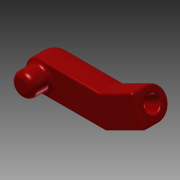
# Autodesk Inventor part: Lego Arm
Saved by Autodesk Inventor 2013 (Build 170138000, 138)
## iProperties
Created: 2013-09-06
Part Number: Lego Arm
Material: Generic
Document SubType Name: Modeling
Designer: 200395375
Density: 1 g/cm^3
Mass: 0.228717 g
Surface Area: 2.72541 cm^2
Volume: 0.228717 cm^3
Author: 200395375
Autodesk Inventor part; units mm, degrees
ref_plane "YZ Plane" through (0, 0, 0) normal (1, 0, 0) x (0, 1, 0)
ref_plane "XZ Plane" through (0, 0, 0) normal (0, 1, 0) x (-1, 0, 0)
ref_plane "XY Plane" through (0, 0, 0) normal (0, 0, 1) x (1, 0, 0)
sketch "Sketch16" plane through (0, 0, 0) normal (0, 1, 0) x (-1, 0, 0)
  circle A0 centre (0, 0) radius 1.5
  dimension "d51" = 3
  constraints: 1 centre point, 1 coincident
  measures "d51" diameter of A0
extrude "Extrusion15" add sketch "Sketch16" along normal blind 2.5
sketch "Sketch17" plane through (0, 2.5, 0) normal (0, 1, 0) x (1, 0, 0)
  line L0 (2, 2) -> (-2, 2)
  line L1 (-2, 2) -> (-2, -2)
  line L2 (-2, -2) -> (2, -2)
  line L3 (2, -2) -> (2, 2)
  dimension "d54" = 4
  dimension "d55" = 4
  constraints: 8 end point, 2 parallel, 1 horizontal, 1 perpendicular
  measures "d54" distance of L2.end L1.end
  measures "d55" distance of L1.end L0.end
extrude "Extrusion16" add sketch "Sketch17" along normal blind 4
sketch "Sketch18" plane through (2, 2.5, 2) normal (1, 0, 0) x (0, 0, -1)
  line L0 (0, 0) -> (4, 0) projected
  line L1 (4, 0) -> (4, 4) projected
  line L2 (0, 4) -> (4, 4) projected
  line L3 (0, 0) -> (0, 4) projected
  point P0 (2, -2.5)
extrude "Extrusion17" add sketch "Sketch18" along normal blind 6
sketch "Sketch21" plane through (0, 6.5, 0) normal (0, 1, 0) x (1, 0, 0)
  line L0 (8, 2) -> (8, -2) projected
  line L1 (8, 2) -> (10, 2)
  line L2 (10, 2) -> (8, -2)
  point P0 (0, 0)
  dimension "d66" = 2
  constraints: 4 end point, 1 perpendicular
  measures "d66" distance of L0.start L1.end
extrude "Extrusion20" add sketch "Sketch21" against normal blind 4
sketch "Sketch22" plane through (8, 2.5, 2) normal (0.8944272, 0, 0.4472136) x (0.4472136, 0, -0.8944272)
  line L0 (4.4721, 0) -> (0, 0) projected
  line L1 (0, 4) -> (4, 4)
  line L2 (4, 4) -> (4, 0)
  line L3 (4, 0) -> (0, 0)
  line L4 (0, 0) -> (0, 4)
  point P0 (-1.7889, -2.5)
  dimension "d69" = 4
  constraints: 8 end point, 2 parallel, 1 horizontal, 1 perpendicular, 1 point on line
  measures "d69" distance of L2.end L3.end
extrude "Extrusion21" add sketch "Sketch22" along normal blind 5
sketch "Sketch23" plane through (0, 6.5, 0) normal (0, 1, 0) x (1, 0, 0)
  line L0 (-2, 2) -> (10, 2) projected
  line L1 (9.7889, 1.5777) -> (10, 2) projected
  line L2 (9.7889, 1.5777) -> (8.9443, 2)
  point P0 (0, 0)
  constraints: 2 end point, 1 perpendicular, 1 point on line
extrude "Extrusion22" cut sketch "Sketch23" against normal blind 5
sketch "Sketch24" plane through (12.4721, 2.5, 4.2361) normal (0.8944272, 0, 0.4472136) x (0.4472136, 0, -0.8944272)
  circle A0 centre (2, 2) radius 1
  point P0 (-1.7889, -2.5)
  dimension "d74" = 2
  constraints: 1 centre point
  measures "d74" diameter of A0
extrude "Extrusion23" cut sketch "Sketch24" against normal blind 2.5
fillet "Fillet7" radius 2 4 edges at (11.6026, 6.5, -0.6708) (3.4721, 6.5, -2) (3, 6.5, 2) (10.2361, 6.5, 3.118)
fillet "Fillet8" radius 2 3 edges at (-2, 5.9142, -1.4142) (-2, 3.5, 2) (-2, 3.5, -2)
fillet "Fillet9" radius 0.25 14 edges at (4.4721, 2.5, -2) (-1.4142, 2.5, 1.4142) (4, 2.5, 2) (11.6026, 2.5, -0.6708) (10.2361, 2.5, 3.118) (13.3666, 2.5, 2.4472) (12.9193, 4.5, 3.3416) (10.6815, 4.5, 2.2227) (8.9443, 3.5, -2) (8.806, 5.9142, -1.4142) (8, 3.5, 2) (14.261, 3.5, 0.6584) (12.4721, 3.5, 4.2361) (13.999, 5.9142, 1.1823)
fillet "Fillet11" radius 0.5 1 edges at (1.5, 2.5, 0)
fillet "Fillet12" radius 0.75 1 edges at (1.5, 0, 0)
body "Solid2"
